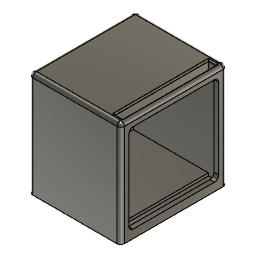
Liphoain BoxV1 (Autodesk Fusion 360 design; units mm, degrees)
Autodesk Fusion 360 part; units mm, degrees
sketch "Sketch1" plane through (0, 0, 0) normal (1, 0, 0) x (0, 1, 0)
  line L0 (51, -51) -> (-51, -51)
  line L1 (-51, -51) -> (-51, 51)
  line L2 (-51, 51) -> (51, 51)
  line L3 (51, 51) -> (51, -51)
  line L4 (51, -51) -> (-51, 51) construction
  line L5 (-51, -51) -> (51, 51) construction
  line L6 (53.5, -53.5) -> (-53.5, -53.5)
  line L7 (-53.5, -53.5) -> (-53.5, 53.5)
  line L8 (-53.5, 53.5) -> (53.5, 53.5)
  line L9 (53.5, 53.5) -> (53.5, -53.5)
  line L10 (53.5, -53.5) -> (-53.5, 53.5) construction
  line L11 (-53.5, -53.5) -> (53.5, 53.5) construction
  line L12 (56, -56) -> (-56, -56)
  line L13 (-56, -56) -> (-56, 56)
  line L14 (-56, 56) -> (56, 56)
  line L15 (56, 56) -> (56, -56)
  line L16 (56, -56) -> (-56, 56) construction
  line L17 (-56, -56) -> (56, 56) construction
  dimension "d1" = 102
  dimension "d2" = 102
  dimension "d3" = 107
  dimension "d4" = 107
  dimension "d5" = 112
  dimension "d6" = 112
  constraint horizontal L0
  constraint perpendicular L0 L1
  constraint parallel L0 L2
  constraint parallel L1 L3
  constraint coincident L4 origin
  constraint coincident L5 origin
  constraint horizontal L6
  constraint perpendicular L6 L7
  constraint parallel L6 L8
  constraint parallel L7 L9
  constraint coincident L10 origin
  constraint coincident L11 origin
  constraint horizontal L12
  constraint perpendicular L12 L13
  constraint parallel L12 L14
  constraint parallel L13 L15
  constraint coincident L16 origin
  constraint coincident L17 origin
  measures "d1" distance of L1.end L2.end
  measures "d2" distance of L0.end L1.end
  measures "d3" distance of L7.end L8.end
  measures "d4" distance of L6.end L7.end
  measures "d5" distance of L13.end L14.end
  measures "d6" distance of L12.end L13.end
extrude "Extrude1" add sketch "Sketch1" along normal blind 100 contours L6 L7 L8 L9 | L12 L13 L14 L15
extrude "Extrude2" add sketch "Sketch1" along normal blind 5 contours L0 L1 L2 L3
sketch "Sketch2" plane through (0, 0, 56) normal (0, 0, 1) x (-1, 0, 0)
  line L0 (0, -56) -> (0, 56)
  line L1 (0, 56) -> (-100, 56)
  line L2 (-100, 56) -> (-100, -56)
  line L3 (-100, -56) -> (0, -56)
  line L4 (-100, 0) -> (-95, 0)
  line L5 (-87, 0) -> (-87, 51)
  line L6 (-87, 51) -> (-95, 51)
  line L7 (-95, 51) -> (-95, 0)
  line L8 (-87, 0) -> (-87, -51)
  line L9 (-87, -51) -> (-95, -51)
  line L10 (-95, -51) -> (-95, 0)
  dimension "d11" = 8
  dimension "d12" = 51
  dimension "d13" = 51
  constraint midpoint L2 L4.start
  constraint perpendicular L2 L4
  constraint vertical L5
  constraint horizontal L6
  constraint vertical L7
  constraint vertical L8
  constraint horizontal L9
  constraint vertical L10
  measures "d11" distance of L4.end L5.start
  measures "d12" distance of L4.end L6.end
  measures "d13" distance of L4.end L9.end
extrude "Extrude3" cut sketch "Sketch2" against normal blind 110 contours L5 L6 L7 L8 L9 L10
extrude "Extrude4" add 1 faces at (96.6667, -17, 51) along direction (0, 0, -1) blind 4
extrude "Extrude5" add 1 faces at (96.6667, 17, -51) along direction (0, 0, 1) blind 4
extrude "Extrude6" cut 1 faces at (96.6667, 17, -47) along direction (0, 0, -1) blind 3
sketch "Sketch3" plane through (0, 51, 0) normal (0, -1, 0) x (1, 0, 0)
  line L0 (100, -50) -> (100, 47)
  line L1 (100, 47) -> (95, 47)
  line L2 (95, 47) -> (95, 56)
  line L3 (95, 56) -> (87, 56)
  line L4 (87, 56) -> (87, 51)
  line L5 (87, 51) -> (5, 51)
  line L6 (5, 51) -> (5, -51)
  line L7 (5, -51) -> (87, -51)
  line L8 (87, -51) -> (87, -54)
  line L9 (87, -54) -> (95, -54)
  line L10 (95, -54) -> (95, -50)
  line L11 (95, -50) -> (100, -50)
  line L12 (95, 47) -> (95, -50)
  constraint coincident L1.end L2.start
  constraint coincident L10.end L11.start
extrude "Extrude7" add sketch "Sketch3" along normal blind 2 contours L0 L1 L11 L12
sketch "Sketch4" plane through (0, -51, 0) normal (0, 1, 0) x (-1, 0, 0)
  line L0 (-95, -50) -> (-95, -54)
  line L1 (-95, -54) -> (-87, -54)
  line L2 (-87, -54) -> (-87, -51)
  line L3 (-87, -51) -> (-5, -51)
  line L4 (-5, -51) -> (-5, 51)
  line L5 (-5, 51) -> (-87, 51)
  line L6 (-87, 51) -> (-87, 56)
  line L7 (-87, 56) -> (-95, 56)
  line L8 (-95, 56) -> (-95, 47)
  line L9 (-95, 47) -> (-100, 47)
  line L10 (-100, 47) -> (-100, -50)
  line L11 (-100, -50) -> (-95, -50)
  line L12 (-95, 47) -> (-95, -50)
  constraint coincident L8.end L9.start
  constraint coincident L0.start L11.end
extrude "Extrude8" add sketch "Sketch4" along normal blind 2 contours L9 L10 L11 L12
extrude "Extrude9" add 1 faces at (33.3333, 18.6667, -56) along direction (0, 0, -1) blind 3
extrude "Extrude10" add 1 faces at (33.3333, 56, 17.6667) along direction (0, 1, 0) blind 2
extrude "Extrude11" add 1 faces at (33.3333, -56, 17.6667) along direction (0, -1, 0) blind 2
fillet "Fillet1" radius 4 4 edges at (50, -58, 56) (50, 58, 56) (100, 0, 56) (0, 0, 56)
fillet "Fillet2" radius 4 8 edges at (100, -58, -3.5) (98.8284, -56.8284, 54.8284) (1.1716, -56.8284, 54.8284) (0, -58, -3.5) (0, 58, -3.5) (1.1716, 56.8284, 54.8284) (98.8284, 56.8284, 54.8284) (100, 58, -3.5)
fillet "Fillet3" radius 1.5 4 edges at (87, 0, 56) (91, 51, 56) (95, 0, 56) (91, -51, 56)
sketch "Sketch5" plane through (0, 0, 51) normal (0, 0, -1) x (1, 0, 0)
  line L0 (87, -51) -> (87, 51)
  line L1 (87, 51) -> (5, 51)
  line L2 (5, 51) -> (5, -51)
  line L3 (5, -51) -> (87, -51)
  line L4 (87, 51) -> (82, 51)
  line L5 (82, 51) -> (82, 51)
  line L6 (82, 51) -> (87, 51)
  line L7 (87, 51) -> (87, 51)
  line L8 (82, -51) -> (87, -51)
  line L9 (87, -51) -> (87, 51)
  line L10 (87, 51) -> (82, 51)
  line L11 (82, 51) -> (82, -51)
  constraint horizontal L4
  constraint horizontal L6
  constraint coincident L1 L4.end
  constraint coincident L0.end L1.start
  constraint horizontal L8
  constraint vertical L9
  constraint horizontal L10
  constraint vertical L11
  constraint coincident L3 L8.start
extrude "Extrude12" add sketch "Sketch5" along normal blind 7 contours L0 L1 L3 L4 L6 L8 L9 L10 L11
fillet "Fillet4" radius 4.5 4 edges at (97.5, 49, 47) (97.5, 49, -50) (97.5, -49, -50) (97.5, -49, 47)
sketch "Sketch6" plane through (5, 0, 0) normal (1, 0, 0) x (0, 1, 0)
  line L0 (51, 51) -> (-51, 51)
  line L1 (-51, 51) -> (-51, -51)
  line L2 (-51, -51) -> (51, -51)
  line L3 (51, -51) -> (51, 51)
  circle A0 centre (0, 0) radius 30
  circle A1 centre (0, 0) radius 2.5
  circle A2 centre (-12.1989, -0.0744) radius 5
  circle A3 centre (12.1996, -0.0472) radius 5
  circle A4 centre (12.1996, -0.0472) radius 1.25
  circle A5 centre (-12.1989, -0.0744) radius 1.25
  line L4 (0, -40) -> (-5, -40)
  line L5 (-5, -40) -> (4.9293, -40)
  line L6 (4.9293, -40) -> (4.9293, -49.4353)
  line L7 (4.9293, -49.4353) -> (-5, -49.4353)
  line L8 (-5, -49.4353) -> (-5, -40)
  dimension "d42" = 60
  dimension "d43" = 5
  dimension "d48" = 10
  dimension "d49" = 10
  dimension "d50" = 2.5
  dimension "d51" = 2.5
  dimension "d52" = 5
  constraint coincident A0.centre A1.centre
  constraint concentric A3 A4
  constraint horizontal L4
  constraint perpendicular L5 L6
  constraint parallel L5 L7
  constraint parallel L6 L8
  constraint parallel L4 L5
  measures "d42" diameter of A0
  measures "d43" diameter of A1
  measures "d48" diameter of A2
  measures "d49" diameter of A3
  measures "d50" diameter of A4
  measures "d51" diameter of A5
  measures "d52" distance of L4.start L4.end
extrude "Extrude14" cut sketch "Sketch6" against normal blind 30 contours L4 L5 L6 L7 L8
fillet "Fillet5" radius 1.5 4 edges at (2.5, 4.9293, -40) (2.5, -5, -40) (2.5, 4.9293, -49.4353) (2.5, -5, -49.4353)
extrude "Extrude15" add 1 faces at (85.3333, 17, 44) along direction (0, 0, -1) blind 1.5
extrude "Extrude16" cut 1 faces at (87, -17, 46.5) along direction (-1, 0, 0) blind 0.2
extrude "Extrude17" cut 1 faces at (87, 17, -53) along direction (-1, 0, 0) blind 0.2
named bodies: "Lithophane Box"
